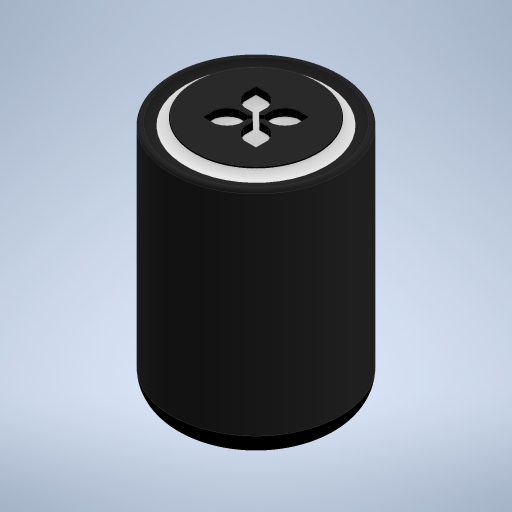
# Autodesk Inventor part: Audio Speaker
Saved by Autodesk Inventor 2024 (Build 280153000, 153)
## iProperties
Created: 2023-07-06
Part Number: Audio Speaker
Material: Generic
Document SubType Name: Modeling
Designer: javie
Density: 1 g/cm^3
Appearance: Default
Author: javie
Autodesk Inventor part; units mm, degrees
ref_plane "YZ Plane" through (0, 0, 0) normal (1, 0, 0) x (0, 1, 0)
ref_plane "XZ Plane" through (0, 0, 0) normal (0, 1, 0) x (-1, 0, 0)
ref_plane "XY Plane" through (0, 0, 0) normal (0, 0, 1) x (1, 0, 0)
sketch "Sketch1" plane through (0, 0, 0) normal (0, 0, 1) x (1, 0, 0)
  line L0 (0, 49.9808) -> (25.2879, 49.9808)
  line L1 (35, 50.0192) -> (35, -39.9808)
  line L2 (25, -49.9808) -> (0, -49.9808)
  line L3 (0, -49.9808) -> (0, 49.9808)
  line L4 (0, 49.9808) -> (0, 0)
  line L5 (21.0691, 46.9303) -> (29.2483, 46.9303)
  arc A0 (29.2483, 46.9303) -> (35, 50.0192) centre (29.2483, 53.8298) ccw
  arc A1 (25.3681, 49.4613) -> (21.0691, 46.9303) centre (28.7319, 38.8314) ccw
  line L6 (0, 93.4458) -> (0, -94.9165) construction
  arc A2 (25.3681, 49.4613) -> (25.2879, 49.9808) centre (25.2879, 49.7149) ccw
  arc A3 (25, -49.9808) -> (35, -39.9808) centre (25, -39.9808) ccw
  point P0 (35, -49.9808)
  dimension "d0" = 35
  dimension "d1" = 100
  dimension "d3" = 10
  constraints: 14 end point, 8 point on circle, 6 tangent, 4 centre point, 2 parallel, 2 perpendicular, 2 point on line, 1 coincident, 1 horizontal, 1 midpoint, 1 vertical
  measures "d0" distance of point (35, -49.981) L2.end
  measures "d1" distance of L1.start point (35, -49.981)
  measures "d3" radius of A3
revolve "Revolution1" add sketch "Sketch1" angle 360 about axis through (0, 93.4458, 0) along (0, -1, 0)
sketch "Sketch2" plane through (0, 49.9808, 0) normal (0, 1, 0) x (1, 0, 0)
  line L0 (-1, 1) -> (-11, 1)
  line L1 (-11, 1) -> (-11, 11)
  line L2 (-11, 11) -> (-1, 11)
  line L3 (-1, 11) -> (-1, 1)
  arc A0 (-11, 6) -> (-6, 1) centre (-4.228, 7.772) ccw
  arc A1 (-1, 6) -> (-6, 11) centre (-7.772, 4.228) ccw
  line L4 (-1, -1) -> (-1, -11)
  line L5 (-1, -11) -> (-11, -11)
  line L6 (-11, -11) -> (-11, -1)
  line L7 (-11, -1) -> (-1, -1)
  arc A2 (-6, -11) -> (-1, -6) centre (-7.772, -4.228) ccw
  arc A3 (-6, -1) -> (-11, -6) centre (-4.228, -7.772) ccw
  line L8 (1, -1) -> (11, -1)
  line L9 (11, -1) -> (11, -11)
  line L10 (11, -11) -> (1, -11)
  line L11 (1, -11) -> (1, -1)
  arc A4 (11, -6) -> (6, -1) centre (4.228, -7.772) ccw
  arc A5 (1, -6) -> (6, -11) centre (7.772, -4.228) ccw
  line L12 (1, 1) -> (1, 11)
  line L13 (1, 11) -> (11, 11)
  line L14 (11, 11) -> (11, 1)
  line L15 (11, 1) -> (1, 1)
  arc A6 (6, 11) -> (1, 6) centre (7.772, 4.228) ccw
  arc A7 (6, 1) -> (11, 6) centre (4.228, 7.772) ccw
  line L16 (1, 2.456) -> (-0.0171, 1.4141)
  line L17 (-1.4141, -0.0171) -> (-2.3736, -1)
  line L18 (2.3736, 1) -> (1.4141, 0.0171)
  line L19 (0.0171, -1.4141) -> (-1, -2.456)
  line L20 (-2.456, 1) -> (-1.4141, -0.0171)
  line L21 (0.0171, -1.4141) -> (1, -2.3736)
  line L22 (-1, 2.3736) -> (-0.0171, 1.4141)
  line L23 (1.4141, 0.0171) -> (2.456, -1)
  point P0 (0, 0)
  point P1 (0, 0)
  dimension "d4" = 10
  dimension "d5" = 10
  dimension "d6" = 1
  dimension "d7" = 1
  dimension "d8" = 7
  dimension "d10" = 7
  dimension "d13" = 360
  constraints: 48 end point, 16 point on circle, 10 parallel, 8 centre point, 8 point on line, 5 perpendicular, 4 midpoint, 1 coincident, 1 horizontal, 65 other
  measures "d4" distance of L1.end L2.end
  measures "d5" distance of L0.end L1.end
  measures "d6" horizontal distance of L0.start point (0, 0)
  measures "d7" distance from line of point (0, 0) L3
  measures "d8" radius of A0
  measures "d10" radius of A1
extrude "Extrusion1" cut sketch "Sketch2" against normal blind 3 contours L3 L22 L16 L12 L15 L18 L23 L8 L11 L21 L19 L4 L7 L17 L20 L0 | L0 A0 L1 L2 A1 L3 | L7 L4 A2 L5 L6 A3 | L12 A6 L13 L14 A7 L15 | L11 L8 A4 L9 L10 A5
fillet "Fillet1" radius 1.25 1 edges at (-35, 50.0192, 0)
body "Solid1"
